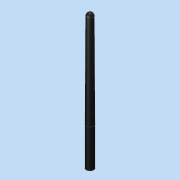
# Autodesk Inventor part: Antenna2
Saved by Autodesk Inventor 2017 (Build 210142000, 142)
## iProperties
Created: 2017-11-03
Part Number: Antenna2
Material: ABS Plastic
Document SubType Name: Modeling
Designer: Derek Wider
Density: 1.06 g/cm^3
Appearance: Glossy - Black
Author: Derek Wider
Autodesk Inventor part; units mm, degrees
ref_plane "YZ Plane" through (0, 0, 0) normal (1, 0, 0) x (0, 1, 0)
ref_plane "XZ Plane" through (0, 0, 0) normal (0, 1, 0) x (-1, 0, 0)
ref_plane "XY Plane" through (0, 0, 0) normal (0, 0, 1) x (1, 0, 0)
sketch "Sketch1" plane through (0, 0, 0) normal (0, 0, 1) x (1, 0, 0)
  line L0 (0, 0) -> (0, 139.7)
  line L1 (0, 0) -> (3.81, 0)
  line L2 (3.81, 0) -> (3.81, 39.2562)
  line L3 (3.81, 39.2562) -> (3.3286, 136.3878)
  arc A0 (3.3286, 136.3878) -> (0, 139.7) centre (0, 136.3713) ccw
  dimension "d0" = 139.7
  dimension "d1" = 3.81
  constraints: 8 end point, 2 point on circle, 1 centre point, 1 horizontal, 1 perpendicular, 1 point on line, 1 tangent, 1 vertical
  measures "d0" distance of L0.start L0.end
  measures "d1" distance of L0.start L1.end
revolve "Revolution1" add sketch "Sketch1" angle 360 about axis through (0, 0, 0) along (0, 1, 0)
body "Solid1"
